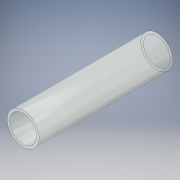
# Autodesk Inventor part: DPLX_P025_Quartz_Tube
Saved by Autodesk Inventor 2018 (Build 220112000, 112)
## iProperties
Created: 2017-11-29
Part Number: DPLX_P025_Quartz_Tube
Material: Glass
Document SubType Name: Modeling
Designer: Pierce
Density: 2.18 g/cm^3
Appearance: Clear
Mass: 30.1342 g
Surface Area: 140.995 cm^2
Volume: 13.823 cm^3
Author: Pierce
Autodesk Inventor part; units mm, degrees
ref_plane "YZ Plane" through (0, 0, 0) normal (1, 0, 0) x (0, 1, 0)
ref_plane "XZ Plane" through (0, 0, 0) normal (0, 1, 0) x (-1, 0, 0)
ref_plane "XY Plane" through (0, 0, 0) normal (0, 0, 1) x (1, 0, 0)
sketch "Sketch1" plane through (0, 0, 0) normal (0, 0, 1) x (1, 0, 0)
  circle A0 centre (0, 0) radius 10
  circle A1 centre (0, 0) radius 12
  dimension "d0" = 20
  dimension "d1" = 2
  constraints: 2 centre point, 1 coincident
  measures "d0" diameter of A0
  measures "d1" radial gap between concentric circles of A0 A1
extrude "Extrusion1" add sketch "Sketch1" along normal mid plane 100
body "Solid1"
